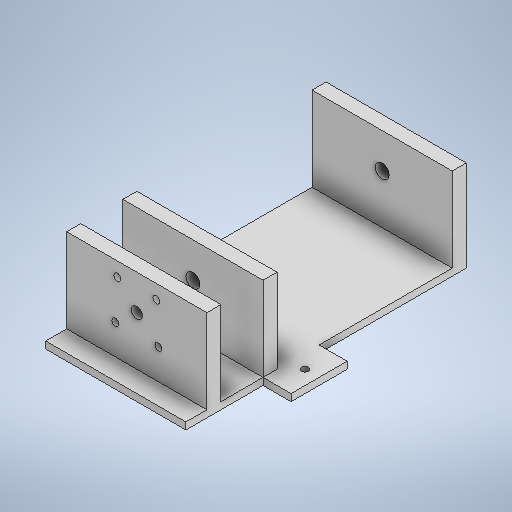
# Autodesk Inventor part: Base_motor
Saved by Autodesk Inventor 2026 (Build 300175050, 175E)
## iProperties
Created: 2025-06-24
Part Number: Base_motor
Material: Genérico
Document SubType Name: Modeling
Designer: piero
Density: 1 g/cm^3
Appearance: Valor por defecto
Author: piero
Autodesk Inventor part; units mm, degrees
ref_plane "YZ Plane" through (0, 0, 0) normal (1, 0, 0) x (0, 1, 0)
ref_plane "XZ Plane" through (0, 0, 0) normal (0, 1, 0) x (-1, 0, 0)
ref_plane "XY Plane" through (0, 0, 0) normal (0, 0, 1) x (1, 0, 0)
sketch "Boceto2" plane through (0, 0, 0) normal (0, 1, 0) x (-1, 0, 0)
  line L0 (0, 0) -> (100, 0)
  line L1 (100, 0) -> (100, -200)
  line L2 (100, -200) -> (0, -200)
  line L3 (0, -200) -> (0, 0)
  dimension "d2" = 200
  dimension "d3" = 100
  constraints: 8 end point, 2 parallel, 1 horizontal, 1 perpendicular
  measures "d2" distance of L0.end L1.end
  measures "d3" distance of L1.end L2.end
extrude "Extrusión1" add sketch "Boceto2" along normal blind 5
sketch "Boceto3" plane through (0, 5, 0) normal (0, 1, 0) x (1, 0, 0)
  line L0 (-100, 200) -> (-100, 0) projected
  line L1 (-100, 55) -> (-120, 55)
  line L2 (-120, 55) -> (-120, 95)
  line L3 (-120, 95) -> (-100, 95)
  line L4 (-100, 95) -> (-100, 55)
  line L5 (0, 0) -> (0, 200) projected
  line L6 (0, 55) -> (20, 55)
  line L7 (20, 55) -> (20, 95)
  line L8 (20, 95) -> (0, 95)
  line L9 (0, 95) -> (0, 55)
  line L10 (-100, 0) -> (0, 0) projected
  circle A0 centre (-110, 75) radius 2.5
  circle A1 centre (10, 75) radius 2.5
  point P0 (0, 95)
  dimension "d6" = 20
  dimension "d7" = 40
  dimension "d8" = 20
  dimension "d9" = 40
  dimension "d10" = 55
  dimension "d11" = 5
  dimension "d12" = 5
  constraints: 16 end point, 4 parallel, 3 point on line, 2 centre point, 2 horizontal, 2 perpendicular
  measures "d6" distance of L2.end L3.end
  measures "d7" distance of L1.end L2.end
  measures "d8" distance of L8.end L7.end
  measures "d9" distance of L7.end L6.end
  measures "d10" distance between parallel lines of L10 L1
  measures "d11" diameter of A0
  measures "d12" diameter of A1
extrude "Extrusión2" add sketch "Boceto3" against normal blind 5
thread "Rosca1" size "M5x0.8" class "6H" standard "ANSI Metric M Profile" full length
thread "Rosca2" size "M5x0.8" class "6H" standard "ANSI Metric M Profile" full length
sketch "Boceto4" plane through (0, 5, 0) normal (0, 1, 0) x (1, 0, 0)
  line L0 (-100, 200) -> (-100, 95) projected
  line L1 (0, 95) -> (0, 200) projected
  line L2 (-100, 200) -> (0, 200)
  line L3 (0, 200) -> (0, 190)
  line L4 (0, 190) -> (-100, 190)
  line L5 (-100, 190) -> (-100, 200)
  line L6 (0, 55) -> (-100, 55)
  line L7 (-100, 55) -> (-100, 65)
  line L8 (-100, 65) -> (0, 65)
  line L9 (0, 65) -> (0, 55)
  line L10 (-100, 15) -> (0, 15)
  line L11 (0, 15) -> (0, 25)
  line L12 (0, 25) -> (-100, 25)
  line L13 (-100, 25) -> (-100, 15)
  line L14 (-100, 0) -> (0, 0) projected
  dimension "d19" = 10
  dimension "d20" = 100
  dimension "d21" = 10
  dimension "d22" = 100
  dimension "d24" = 30
  dimension "d56" = 125
  constraints: 24 end point, 6 parallel, 3 horizontal, 3 perpendicular, 2 point on line
  measures "d19" distance between parallel lines of L2 L4
  measures "d20" distance of L7.end L8.end
  measures "d21" distance of L6.end L7.end
  measures "d22" distance of L12.end L11.end
  measures "d24" distance between parallel lines of L6 L12
  measures "d56" distance between parallel lines of L4 L8
extrude "Extrusión3" add sketch "Boceto4" along normal blind 60
sketch "Boceto5" plane through (0, 0, -200) normal (0, 0, -1) x (-1, 0, 0)
  circle A0 centre (50, 40) radius 5
  line L0 (0, 0) -> (0, 65) projected
  line L1 (0, 0) -> (100, 0) projected
  dimension "d28" = 10
  dimension "d29" = 50
  dimension "d34" = 40
  constraints: 1 centre point
  measures "d28" diameter of A0
  measures "d29" distance from line of A0.centre L0
  measures "d34" distance from line of L1 A0.centre
extrude "Extrusión4" cut sketch "Boceto5" against normal blind 10
sketch "Boceto6" plane through (0, 5, -65) normal (0, 0, -1) x (-1, 0, 0)
  circle A0 centre (50, 35) radius 5 projected
  circle A1 centre (50, 35) radius 5
  point P0 (0, -5)
  constraints: 1 centre point, 1 coincident
extrude "Extrusión5" cut sketch "Boceto6" against normal blind 10
sketch "Boceto7" plane through (-100, 5, -15) normal (0, 0, 1) x (1, 0, 0)
  circle A0 centre (50, 35) radius 5 projected
  circle A1 centre (50, 35) radius 4
  circle A2 centre (36.1091, 50) radius 2.5
  circle A3 centre (63.8909, 50) radius 2.5
  line L0 (0, 0) -> (0, 60) projected
  line L1 (100, 0) -> (100, 60) projected
  circle A4 centre (34.6472, 21.5) radius 2.5
  circle A5 centre (65.3528, 21.5) radius 2.5
  line L2 (0, 60) -> (100, 60) projected
  line L3 (0, 0) -> (100, 0) projected
  point P0 (100, -5)
  dimension "d35" = 8
  dimension "d36" = 5
  dimension "d37" = 5
  dimension "d41" = 5
  dimension "d42" = 5
  dimension "d45" = 10
  dimension "d47" = 10
  dimension "d50" = 20.444
  dimension "d51" = 28.5
  dimension "d52" = 20.444
  dimension "d53" = 20.444
  dimension "d54" = 20.444
  dimension "d55" = 28.5
  constraints: 5 centre point, 1 coincident
  measures "d35" diameter of A1
  measures "d36" diameter of A2
  measures "d37" diameter of A3
  measures "d41" diameter of A4
  measures "d42" diameter of A5
  measures "d45" distance from line of L2 A2.centre
  measures "d47" distance from line of A3.centre L2
  measures "d50" distance of A1.centre A2.centre
  measures "d51" vertical distance of A2.centre A4.centre
  measures "d52" distance of A1.centre A4.centre
  measures "d53" distance of A1.centre A3.centre
  measures "d54" distance of A1.centre A5.centre
  measures "d55" vertical distance of A5.centre A3.centre
extrude "Extrusión6" cut sketch "Boceto7" against normal blind 10 contours A1 | A2 | A3 | A4 | A5
